Autodesk Fusion 360 part; units mm, degrees
note: some values were not read from the file. Chosen so that the rebuilt part matches the saved one: which bodies a step acts on; which face or edge a step refers to. Set by a fixed rule: which sketch regions a step uses.
(part 2 of 2)
  dimension "d542" = 3
  dimension "d543" = 3
  dimension "d544" = 3
  dimension "d545" = 3
  dimension "d571" = 15
  dimension "d572" = 30
  dimension "d573" = 15
  dimension "d574" = 30
  dimension "d575" = 30
  dimension "d576" = 5.5
  dimension "d578" = 30
  dimension "d579" = 5
  dimension "d580" = 5
  dimension "d581" = 5
  dimension "d582" = 5
  dimension "d583" = 15
  dimension "d584" = 30
  dimension "d585" = 30
  dimension "d586" = 15
  dimension "d587" = 30
  dimension "d588" = 5.5
  dimension "d591" = 30
  dimension "d592" = 5
  dimension "d593" = 5
  dimension "d594" = 5
  dimension "d595" = 5
  constraint perpendicular L3 L20
  constraint tangent A0 L2
  constraint tangent A0 L21
  constraint tangent L1 A13
  constraint tangent L21 A13
  constraint tangent A3 L3
  constraint tangent A3 L20
  constraint tangent L8 A8
  constraint tangent A8 L20
  constraint tangent L16 A782
  constraint tangent L9 A782
  constraint tangent L6 A783
  constraint tangent L9 A783
  constraint tangent L12 A784
  constraint tangent L13 A784
  constraint tangent L10 A785
  constraint tangent L13 A785
  constraint tangent L0 A786
  constraint tangent L18 A786
  constraint tangent L18 A787
  constraint tangent L19 A787
  constraint tangent L4 A788
  constraint tangent L15 A788
  constraint tangent L5 A789
  constraint tangent L4 A789
  constraint parallel L7 L23
  constraint perpendicular L6 L24
  constraint perpendicular L10 L25
  constraint tangent L25 A791
  constraint coincident L10.start A791.start
  constraint tangent L24 A792
  constraint coincident L12.end A792.end
  constraint tangent L24 A793
  constraint coincident L6.start A793.start
  constraint tangent L23 A794
  constraint coincident L16.end A794.end
  constraint parallel L3 L26
  constraint perpendicular L0 L28
  constraint tangent L28 A796
  constraint coincident L0.end A796.start
  constraint tangent L27 A797
  constraint coincident L19.start A797.end
  constraint tangent L27 A798
  constraint coincident L15.end A798.start
  constraint tangent L26 A799
  constraint coincident L5.start A799.end
  measures "d1" diameter of A12
  measures "d4" radius of A0
  measures "d5" radius of A13
  measures "d6" radius of A3
  measures "d7" radius of A8
  measures "d116" distance of A17.centre A14.centre
  measures "d152" distance of A14.centre A17.centre
  measures "d227" distance of A14.centre A17.centre
  measures "d230" distance of A14.centre A17.centre
  measures "d232" distance of L20 L21
  measures "d303" distance of A14.centre A17.centre
  measures "d305" distance of A16.centre A15.centre
  measures "d306" distance of A14.centre A17.centre
  measures "d310" distance of A14.centre A17.centre
  measures "d313" distance of A14.centre A17.centre
  measures "d319" vertical distance of A14.centre A15.centre
  measures "d448" distance of A494.centre A430.centre
  measures "d449" distance of A494.centre A430.centre
  measures "d450" distance of A494.centre A430.centre
  measures "d451" distance of A494.centre A430.centre
  measures "d452" distance of A494.centre A430.centre
  measures "d453" distance of A432.centre A473.centre
  measures "d454" distance of A430.centre A494.centre
  measures "d455" distance of A430.centre A494.centre
  measures "d456" distance of A494.centre A430.centre
  measures "d457" vertical distance of A494.centre A432.centre
  measures "d459" distance of L20 A56.centre
  measures "d460" distance of L21 A428.centre
  measures "d461" vertical distance of A53.centre A427.centre
  measures "d538" radius of A782
  measures "d539" radius of A783
  measures "d540" radius of A784
  measures "d541" radius of A785
  measures "d542" radius of A786
  measures "d543" radius of A787
  measures "d544" radius of A788
  measures "d545" radius of A789
  measures "d571" distance of A10.centre L21
  measures "d572" distance of A9.centre A10.centre
  measures "d573" distance of A6.centre L20
  measures "d574" distance of A11.centre A6.centre A430.centre
  measures "d575" distance of A9.centre A1.centre A430.centre
  measures "d576" diameter of A790
  measures "d578" distance of A11.centre A790.centre
  measures "d579" radius of A791
  measures "d580" radius of A792
  measures "d581" radius of A793
  measures "d582" radius of A794
  measures "d583" distance of A2.centre L21
  measures "d584" distance of A2.centre A4.centre
  measures "d585" distance of A5.centre A4.centre
  measures "d586" distance of A12.centre L22
  measures "d587" distance of A12.centre A7.centre
  measures "d588" diameter of A795
  measures "d591" distance of A5.centre A795.centre
  measures "d592" radius of A796
  measures "d593" radius of A797
  measures "d594" radius of A798
  measures "d595" radius of A799
extrude "Extrude1" add sketch "Sketch1" along normal blind 3 contours A0 L0 L1 A3 L2 L3 L4 L5 L6 L7 L8 A8 L9 L10 L11 L12 L13 L15 L16 L18 L19 L20 L21 A13 L22 A782 A783 A784 A785 A786 A787 A788 A789 L23 L24 L25 A791 A792 A793 A794 L26 L27 L28 A796 A797 A798 A799 | A14 A18 A26 A29 A66 A73 A87 A88 A115 A123 A124 A130 A134 A154 A174 A191 A250 A254 A306 A313 A323 A326 A328 A337 A338 A339 A340 A345 A347 A348 A364 A380 | A15 A20 A22 A27 A64 A65 A77 A83 A129 A131 A138 A159 A171 A176 A193 A200 A222 A226 A232 A234 A235 A245 A261 A277 A285 A289 A295 A310 A357 A376 A381 A385 | A16 A19 A24 A28 A68 A72 A105 A109 A121 A127 A136 A156 A158 A166 A184 A190 A247 A251 A255 A256 A263 A264 A276 A283 A293 A307 A314 A319 A320 A336 A359 A383 | A17 A21 A23 A25 A69 A86 A92 A102 A128 A133 A155 A167 A180 A182 A197 A202 A219 A220 A221 A227 A230 A241 A257 A260 A270 A279 A291 A369 A371 A386 A387 A394 | A30 A93 A126 A169 A267 A312 A316 A389 | A31 A84 A151 A163 A215 A290 A362 A395 | A32 A104 A157 A195 A233 A294 A365 A374 | A33 A82 A116 A147 A262 A288 A324 A325 | A34 A71 A120 A185 A259 A265 A309 A317 | A35 A90 A140 A173 A206 A210 A212 A213 | A36 A67 A118 A139 A207 A208 A297 A299 | A37 A108 A114 A122 A209 A211 A296 A300 | A38 A96 A150 A204 A266 A382 A384 A390 | A39 A97 A144 A179 A268 A287 A366 A373 | A40 A91 A145 A177 A282 A358 A372 A379 | A41 A70 A132 A188 A253 A305 A311 A333 | A42 A89 A189 A196 A273 A274 A286 A363 | A43 A79 A153 A199 A301 A302 A341 A342 | A44 A95 A152 A201 A303 A304 A331 A349 | A45 A80 A141 A175 A284 A308 A315 A344 | A46 A103 A119 A178 A223 A321 A329 A355 | A47 A106 A165 A203 A249 A281 A334 A346 | A48 A107 A162 A192 A236 A278 A327 A354 | A49 A78 A187 A198 A280 A332 A335 A367 | A50 A63 A117 A142 A318 A322 A330 A343 | A51 A81 A183 A186 A214 A217 A298 A353 | A52 A75 A135 A143 A224 A225 A231 A350 | A53 A76 A137 A146 A216 A239 A351 A352 | A54 A99 A110 A112 A246 A361 A377 A396 | A55 A101 A113 A168 A218 A237 A240 A388 | A56 A98 A111 A164 A229 A370 A392 A397 | A57 A94 A125 A205 A228 A244 A356 A391 | A58 A74 A148 A170 A242 A243 A252 A275 | A59 A85 A149 A161 A258 A269 A360 A375 | A60 A100 A181 A194 A272 A292 A368 A378 | A61 A62 A160 A172 A238 A248 A271 A393 | A398 A416 A419 A421 A569 A574 A645 A747 | A399 A409 A575 A644 A658 A661 A671 A775 | A400 A402 A404 A406 A418 A420 A426 A572 | A401 A403 A405 A411 A412 A423 A571 A776 | A407 A408 A422 A570 A573 A641 A646 A748 | A410 A414 A417 A750 A774 A777 A779 A781 | A413 A424 A567 A576 A640 A751 A752 A780 | A415 A425 A568 A649 A653 A749 A753 A778 | A427 A435 A437 A438 A551 A694 A721 A728 | A428 A431 A517 A519 A690 A692 A706 A731 | A429 A443 A445 A452 A542 A561 A718 A744 | A430 A434 A442 A447 A449 A451 A472 A508 A521 A525 A531 A540 A541 A545 A548 A550 A563 A566 A678 A681 A691 A696 A701 A703 A708 A712 A715 A720 A723 A724 A735 A743 | A432 A444 A446 A471 A480 A484 A489 A490 A493 A495 A511 A512 A515 A520 A530 A533 A579 A597 A598 A682 A683 A685 A693 A697 A707 A711 A716 A719 A729 A732 A733 A737 | A433 A440 A448 A677 A722 A734 A742 A746 | A436 A513 A534 A535 A537 A679 A686 A738 | A439 A441 A547 A553 A554 A555 A556 A560 | A450 A475 A498 A522 A689 A698 A709 A726 | A453 A454 A462 A465 A651 A659 A664 A673 | A455 A458 A464 A467 A470 A543 A549 A565 | A456 A457 A469 A656 A657 A663 A668 A669 | A459 A463 A466 A559 A643 A648 A660 A670 | A460 A544 A546 A552 A557 A558 A562 A564 | A461 A468 A652 A662 A666 A672 A674 A675 | A473 A476 A477 A485 A496 A497 A501 A503 A504 A518 A523 A527 A529 A532 A538 A582 A586 A588 A594 A599 A684 A688 A699 A700 A704 A705 A710 A713 A714 A727 A730 A745 | A474 A487 A502 A578 A589 A619 A631 A639 | A478 A486 A506 A516 A536 A581 A587 A601 | A479 A481 A483 A505 A577 A580 A627 A635 | A482 A491 A500 A526 A528 A583 A592 A600 | A488 A499 A584 A585 A590 A591 A595 A596 | A492 A507 A509 A510 A514 A524 A539 A687 | A494 A602 A603 A604 A605 A606 A607 A609 A610 A612 A613 A617 A618 A621 A622 A623 A624 A626 A629 A630 A633 A634 A636 A637 A638 A702 A758 A759 A761 A767 A769 A771 | A593 A608 A611 A616 A620 A628 A757 A772 | A614 A615 A632 A755 A756 A762 A763 A766 | A625 A754 A760 A764 A765 A768 A770 A773 | A642 A647 A650 A654 A655 A665 A667 A676 | A680 A695 A717 A725 A736 A739 A740 A741 | A790 | A795 makes body 1
sketch "Sketch2" plane through (0, 3, 0) normal (0, 1, 0) x (-1, 0, 0)
  circle A0 centre (-15, -105) radius 2.75
  circle A1 centre (-184, -165) radius 2.75
  circle A2 centre (-184, -135) radius 2.75
  circle A3 centre (-184, -105) radius 2.75
  circle A4 centre (-15, -15) radius 2.75
  circle A5 centre (-184, -45) radius 2.75
  circle A6 centre (-15, -135) radius 2.75
  circle A7 centre (-15, -165) radius 2.75
  circle A8 centre (-15, -45) radius 2.75
  circle A9 centre (-184, -15) radius 2.75
  line L0 (-28, -115) -> (-5, -115)
  line L1 (0, -110) -> (0, -70)
  line L2 (-5, -65) -> (-28, -65)
  line L3 (-31, -62) -> (-31, -58)
  line L4 (-28, -55) -> (-5, -55)
  line L5 (0, -50) -> (0, -10)
  arc A10 (0, -10) -> (-10, 0) centre (-10, -10) ccw
  line L6 (-10, 0) -> (-189, 0)
  arc A11 (-189, 0) -> (-199, -10) centre (-189, -10) ccw
  line L7 (-199, -10) -> (-199, -50)
  line L8 (-194, -55) -> (-171, -55)
  line L9 (-168, -58) -> (-168, -62)
  line L10 (-171, -65) -> (-194, -65)
  line L11 (-194, -115) -> (-171, -115)
  line L12 (-168, -118) -> (-168, -122)
  line L13 (-171, -125) -> (-194, -125)
  line L14 (-199, -130) -> (-199, -170)
  arc A12 (-199, -170) -> (-189, -180) centre (-189, -170) ccw
  line L15 (-189, -180) -> (-10, -180)
  arc A13 (-10, -180) -> (0, -170) centre (-10, -170) ccw
  line L16 (0, -170) -> (0, -130)
  line L17 (-5, -125) -> (-28, -125)
  line L18 (-31, -122) -> (-31, -118)
  circle A14 centre (-50, -40) radius 10
  circle A15 centre (-50, -140) radius 10
  circle A16 centre (-110, -140) radius 10
  circle A17 centre (-110, -90) radius 12.5
  circle A18 centre (-110, -40) radius 10
  circle A19 centre (-160, -90) radius 1.75
  circle A20 centre (-150, -90) radius 1.75
  circle A21 centre (-140, -90) radius 1.75
  circle A22 centre (-130, -90) radius 1.75
  circle A23 centre (-90, -90) radius 1.75
  circle A24 centre (-80, -90) radius 1.75
  circle A25 centre (-70, -90) radius 1.75
  circle A26 centre (-60, -90) radius 1.75
  circle A27 centre (-50, -90) radius 1.75
  line L19 (-10, 0) -> (-189, 0)
  line L20 (0, -60) -> (0, -30)
  line L21 (0, -142) -> (0, -128.1084)
  line L22 (-10, -180) -> (-189, -180)
  circle A28 centre (-99.8, -157.5) radius 1.75
  circle A29 centre (-122.8, -157.5) radius 1.75
  circle A30 centre (-121.5, -122.5) radius 1.75
  circle A31 centre (-98.5, -122.5) radius 1.75
  arc A32 (-168, -58) -> (-171, -55) centre (-171, -58) ccw
  arc A33 (-171, -65) -> (-168, -62) centre (-171, -62) ccw
  arc A34 (-168, -118) -> (-171, -115) centre (-171, -118) ccw
  arc A35 (-171, -125) -> (-168, -122) centre (-171, -122) ccw
  arc A36 (-31, -122) -> (-28, -125) centre (-28, -122) ccw
  arc A37 (-28, -115) -> (-31, -118) centre (-28, -118) ccw
  arc A38 (-31, -62) -> (-28, -65) centre (-28, -62) ccw
  arc A39 (-28, -55) -> (-31, -58) centre (-28, -58) ccw
  circle A40 centre (-98.5, -57.5) radius 1.75
  circle A41 centre (-120.2, -22.5) radius 1.75
  circle A42 centre (-97.2, -22.5) radius 1.75
  circle A43 centre (-121.5, -57.5) radius 1.75
  arc A44 (-199, -50) -> (-194, -55) centre (-194, -50) ccw
  arc A45 (-194, -65) -> (-199, -70) centre (-194, -70) ccw
  line L23 (-199, -70) -> (-199, -110)
  arc A46 (-199, -110) -> (-194, -115) centre (-194, -110) ccw
  arc A47 (-194, -125) -> (-199, -130) centre (-194, -130) ccw
  arc A48 (0, -130) -> (-5, -125) centre (-5, -130) ccw
  arc A49 (-5, -115) -> (0, -110) centre (-5, -110) ccw
  arc A50 (0, -70) -> (-5, -65) centre (-5, -70) ccw
  arc A51 (-5, -55) -> (0, -50) centre (-5, -50) ccw
  point P0 (-63, -24)
  point P1 (-63, -24)
  point P2 (-64.3, -156)
  point P3 (-63, -121.74)
  dimension "d468" = 20
  dimension "d472" = 20
  dimension "d477" = 20
  dimension "d478" = 25
  dimension "d479" = 20
  dimension "d480" = 50
  dimension "d483" = 3.5
  dimension "d486" = 30
  dimension "d487" = 0
  dimension "d488" = 3.5
  dimension "d491" = 40
  dimension "d492" = 0
  dimension "d508" = 50
  dimension "d509" = 50
  dimension "d513" = 40
  dimension "d514" = 40
  dimension "d515" = 3.5
  dimension "d516" = 3.5
  dimension "d517" = 3.5
  dimension "d518" = 3.5
  dimension "d519" = 23
  dimension "d520" = 23
  dimension "d521" = 35
  dimension "d522" = 35
  dimension "d556" = 3.5
  dimension "d557" = 3.5
  dimension "d558" = 3.5
  dimension "d559" = 3.5
  dimension "d560" = 23
  dimension "d561" = 23
  dimension "d562" = 35
  dimension "d563" = 35
  dimension "d564" = 11.5
  dimension "d565" = 17.5
  dimension "d567" = 11.5
  dimension "d568" = 17.5
  measures "d468" diameter of A14
  measures "d472" diameter of A15
  measures "d477" diameter of A16
  measures "d478" diameter of A17
  measures "d479" diameter of A18
  measures "d480" distance of A17.centre A18.centre
  measures "d483" diameter of A19
  measures "d488" diameter of A23
  measures "d508" distance of A14.centre L20
  measures "d509" distance of A15.centre L21
  measures "d513" distance of A14.centre L19
  measures "d514" distance of A15.centre L22
  measures "d515" diameter of A28
  measures "d516" diameter of A29
  measures "d517" diameter of A31
  measures "d518" diameter of A30
  measures "d519" distance of A28.centre A29.centre
  measures "d520" horizontal distance of A30.centre A31.centre
  measures "d521" vertical distance of A29.centre A30.centre
  measures "d522" vertical distance of A28.centre A31.centre
  measures "d556" diameter of A40
  measures "d557" diameter of A43
  measures "d558" diameter of A42
  measures "d559" diameter of A41
  measures "d560" distance of A40.centre A43.centre
  measures "d561" horizontal distance of A42.centre A41.centre
  measures "d562" vertical distance of A43.centre A41.centre
  measures "d563" vertical distance of A40.centre A42.centre
  measures "d564" horizontal distance of A16.centre A30.centre
  measures "d565" vertical distance of A16.centre A28.centre
  measures "d567" horizontal distance of A18.centre A43.centre
  measures "d568" vertical distance of A18.centre A43.centre
extrude "Extrude2" cut sketch "Sketch2" against normal blind 3 contours A14 bodies 1
extrude "Extrude4" cut sketch "Sketch2" against normal blind 3 contours A15 bodies 1
extrude "Extrude5" cut sketch "Sketch2" against normal blind 3 contours A16 | A17 | A18 bodies 1
extrude "Extrude6" cut sketch "Sketch2" against normal blind 3 contours A19 | A20 | A21 | A22 | A23 | A24 | A25 | A26 | A27 bodies 1
extrude "Extrude7" add sketch "Sketch2" against normal blind 3 contours A14 bodies 1
extrude "Extrude8" add sketch "Sketch2" against normal blind 3 contours A15 bodies 1
extrude "Extrude9" cut sketch "Sketch2" against normal blind 3 contours A14 | A15 | A28 | A29 | A30 | A31 bodies 1
extrude "Extrude10" cut sketch "Sketch1" along normal blind 3 contours A14 A18 A26 A29 A66 A73 A87 A88 A115 A123 A124 A130 A134 A154 A174 A191 A250 A254 A306 A313 A323 A326 A328 A337 A338 A339 A340 A345 A347 A348 A364 A380 | A15 A20 A22 A27 A64 A65 A77 A83 A129 A131 A138 A159 A171 A176 A193 A200 A222 A226 A232 A234 A235 A245 A261 A277 A285 A289 A295 A310 A357 A376 A381 A385 | A16 A19 A24 A28 A68 A72 A105 A109 A121 A127 A136 A156 A158 A166 A184 A190 A247 A251 A255 A256 A263 A264 A276 A283 A293 A307 A314 A319 A320 A336 A359 A383 | A17 A21 A23 A25 A69 A86 A92 A102 A128 A133 A155 A167 A180 A182 A197 A202 A219 A220 A221 A227 A230 A241 A257 A260 A270 A279 A291 A369 A371 A386 A387 A394 | A30 A93 A126 A169 A267 A312 A316 A389 | A31 A84 A151 A163 A215 A290 A362 A395 | A32 A104 A157 A195 A233 A294 A365 A374 | A33 A82 A116 A147 A262 A288 A324 A325 | A34 A71 A120 A185 A259 A265 A309 A317 | A35 A90 A140 A173 A206 A210 A212 A213 | A36 A67 A118 A139 A207 A208 A297 A299 | A37 A108 A114 A122 A209 A211 A296 A300 | A38 A96 A150 A204 A266 A382 A384 A390 | A39 A97 A144 A179 A268 A287 A366 A373 | A40 A91 A145 A177 A282 A358 A372 A379 | A41 A70 A132 A188 A253 A305 A311 A333 | A42 A89 A189 A196 A273 A274 A286 A363 | A43 A79 A153 A199 A301 A302 A341 A342 | A44 A95 A152 A201 A303 A304 A331 A349 | A45 A80 A141 A175 A284 A308 A315 A344 | A46 A103 A119 A178 A223 A321 A329 A355 | A47 A106 A165 A203 A249 A281 A334 A346 | A48 A107 A162 A192 A236 A278 A327 A354 | A49 A78 A187 A198 A280 A332 A335 A367 | A50 A63 A117 A142 A318 A322 A330 A343 | A51 A81 A183 A186 A214 A217 A298 A353 | A52 A75 A135 A143 A224 A225 A231 A350 | A53 A76 A137 A146 A216 A239 A351 A352 | A54 A99 A110 A112 A246 A361 A377 A396 | A55 A101 A113 A168 A218 A237 A240 A388 | A56 A98 A111 A164 A229 A370 A392 A397 | A57 A94 A125 A205 A228 A244 A356 A391 | A58 A74 A148 A170 A242 A243 A252 A275 | A59 A85 A149 A161 A258 A269 A360 A375 | A60 A100 A181 A194 A272 A292 A368 A378 | A61 A62 A160 A172 A238 A248 A271 A393 | A398 A416 A419 A421 A569 A574 A645 A747 | A399 A409 A575 A644 A658 A661 A671 A775 | A400 A402 A404 A406 A418 A420 A426 A572 | A401 A403 A405 A411 A412 A423 A571 A776 | A407 A408 A422 A570 A573 A641 A646 A748 | A410 A414 A417 A750 A774 A777 A779 A781 | A413 A424 A567 A576 A640 A751 A752 A780 | A415 A425 A568 A649 A653 A749 A753 A778 | A427 A435 A437 A438 A551 A694 A721 A728 | A428 A431 A517 A519 A690 A692 A706 A731 | A429 A443 A445 A452 A542 A561 A718 A744 | A430 A434 A442 A447 A449 A451 A472 A508 A521 A525 A531 A540 A541 A545 A548 A550 A563 A566 A678 A681 A691 A696 A701 A703 A708 A712 A715 A720 A723 A724 A735 A743 | A432 A444 A446 A471 A480 A484 A489 A490 A493 A495 A511 A512 A515 A520 A530 A533 A579 A597 A598 A682 A683 A685 A693 A697 A707 A711 A716 A719 A729 A732 A733 A737 | A433 A440 A448 A677 A722 A734 A742 A746 | A436 A513 A534 A535 A537 A679 A686 A738 | A439 A441 A547 A553 A554 A555 A556 A560 | A450 A475 A498 A522 A689 A698 A709 A726 | A453 A454 A462 A465 A651 A659 A664 A673 | A455 A458 A464 A467 A470 A543 A549 A565 | A456 A457 A469 A656 A657 A663 A668 A669 | A459 A463 A466 A559 A643 A648 A660 A670 | A460 A544 A546 A552 A557 A558 A562 A564 | A461 A468 A652 A662 A666 A672 A674 A675 | A473 A476 A477 A485 A496 A497 A501 A503 A504 A518 A523 A527 A529 A532 A538 A582 A586 A588 A594 A599 A684 A688 A699 A700 A704 A705 A710 A713 A714 A727 A730 A745 | A474 A487 A502 A578 A589 A619 A631 A639 | A478 A486 A506 A516 A536 A581 A587 A601 | A479 A481 A483 A505 A577 A580 A627 A635 | A482 A491 A500 A526 A528 A583 A592 A600 | A488 A499 A584 A585 A590 A591 A595 A596 | A492 A507 A509 A510 A514 A524 A539 A687 | A494 A602 A603 A604 A605 A606 A607 A609 A610 A612 A613 A617 A618 A621 A622 A623 A624 A626 A629 A630 A633 A634 A636 A637 A638 A702 A758 A759 A761 A767 A769 A771 | A593 A608 A611 A616 A620 A628 A757 A772 | A614 A615 A632 A755 A756 A762 A763 A766 | A625 A754 A760 A764 A765 A768 A770 A773 | A642 A647 A650 A654 A655 A665 A667 A676 | A680 A695 A717 A725 A736 A739 A740 A741 bodies 1
sketch "Sketch3" plane through (99.5, 0, -90) normal (0, 1, 0) x (1, 0, 0)
  line L0 (68.5, 90) -> (73.5, 90)
  line L1 (73.5, 90) -> (73.5, -90)
  line L2 (73.5, -90) -> (68.5, -90)
  line L3 (68.5, -90) -> (68.5, 90)
  line L4 (99.5, 60) -> (99.5, 25)
  line L5 (-68.5, 90) -> (-73.5, 90)
  line L6 (-73.5, 90) -> (-73.5, -90)
  line L7 (-73.5, -90) -> (-68.5, -90)
  line L8 (-68.5, -90) -> (-68.5, 90)
  line L9 (-99.5, 60) -> (-99.5, 22)
  dimension "d531" = 5
  dimension "d532" = 31
  dimension "d533" = 5
  dimension "d534" = 31
  constraint horizontal L0
  constraint vertical L1
  constraint horizontal L2
  constraint vertical L3
  constraint horizontal L5
  constraint vertical L6
  constraint horizontal L7
  constraint vertical L8
  measures "d531" distance of L1 L3
  measures "d532" distance of L3 L4
  measures "d533" distance of L6 L8
  measures "d534" distance of L8 L9
extrude "Extrude11" cut sketch "Sketch3" along normal blind 2 bodies 1
extrude "Extrude12" cut sketch "Sketch2" against normal blind 3 contours A28 | A29 | A30 | A31 | A40 | A41 | A42 | A43 bodies 1
extrude "Extrude13" cut sketch "Sketch1" along normal blind 3 contours A790 | A795 bodies 1
split "Split1" by plane through (168, 0, -118) normal (1, 0, 0) bodies 1 makes body 2 at (172.9668, 3, -23.8898) makes body 3 at (194.672, 3, -85.6235) makes body 4 at (172.9668, 3, -156.1102)
split "Split2" by plane through (31, 0, -118) normal (-1, 0, 0) bodies 1 makes body 5 at (4.328, 3, -85.6235) makes body 6 at (26.0332, 3, -156.1102) makes body 7 at (26.0332, 3, -23.8898)
move_body "Move1" bodies 2 3 4 to x (0, 1, 0) y (-1, 0, 0) z (0, 0, 1) at (171, -168, 0)
move_body "Move2" bodies 7 5 6 to x (0, -1, 0) y (1, 0, 0) z (0, 0, 1) at (28, 31, 0)
extrude "Extrude3" [suppressed]

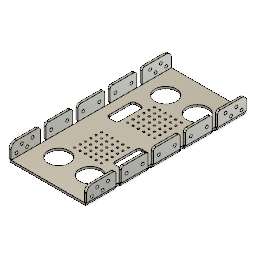
design "Trunk Bottom 4mm"
Autodesk Fusion 360 part; units mm, degrees
sketch "Sketch1" plane through (0, 0, 0) normal (0, 1, 0) x (1, 0, 0)
  line L0 (10, 0) -> (189, 0)
  line L1 (189, 300) -> (10, 300)
  circle A0 centre (184, 165) radius 2.75
  circle A1 centre (184, 135) radius 2.75
  circle A2 centre (184, 195) radius 2.75
  circle A3 centre (184, 105) radius 2.75
  arc A4 (10, 300) -> (0, 290) centre (10, 290) ccw
  arc A5 (199, 290) -> (189, 300) centre (189, 290) ccw
  arc A6 (0, 10) -> (10, 0) centre (10, 10) ccw
  arc A7 (189, 0) -> (199, 10) centre (189, 10) ccw
  circle A8 centre (184, 225) radius 2.75
  line L2 (199, 232.541) -> (199, 232)
  line L3 (199, 202) -> (199, 215)
  line L4 (199, 282) -> (199, 290)
  line L5 (194, 175) -> (171, 175)
  line L6 (171, 185) -> (194, 185)
  line L7 (168, 178) -> (168, 182)
  line L8 (194, 115) -> (171, 115)
  line L9 (171, 125) -> (194, 125)
  line L10 (168, 118) -> (168, 122)
  line L11 (0, 290) -> (0, 270)
  line L12 (0, 68.1084) -> (0, 68)
  line L13 (0, 30) -> (0, 10)
  line L14 (199, 10) -> (199, 30)
  line L15 (199, 85) -> (199, 98)
  line L16 (0, 52) -> (0, 52.1084)
  line L17 (0, 112) -> (0, 112.1084)
  line L18 (0, 142) -> (0, 142.1084)
  line L19 (0, 172) -> (0, 172.1084)
  line L20 (0, 202) -> (0, 202.1084)
  line L21 (0, 232) -> (0, 232.1084)
  line L22 (0, 262) -> (0, 262.1084)
  circle A9 centre (15, 105) radius 2.75
  circle A10 centre (15, 135) radius 2.75
  circle A11 centre (15, 165) radius 2.75
  circle A12 centre (15, 195) radius 2.75
  circle A13 centre (15, 225) radius 2.75
  line L23 (5, 115) -> (28, 115)
  line L24 (28, 125) -> (5, 125)
  line L25 (31, 118) -> (31, 122)
  line L26 (28, 185) -> (5, 185)
  line L27 (5, 175) -> (28, 175)
  line L28 (31, 178) -> (31, 182)
  circle A14 centre (10, 280) radius 2.75
  circle A15 centre (20, 270) radius 2.75
  circle A16 centre (20, 290) radius 2.75
  circle A17 centre (20, 30) radius 2.75
  circle A18 centre (10, 20) radius 2.75
  circle A19 centre (20, 10) radius 2.75
  circle A20 centre (179, 10) radius 2.75
  circle A21 centre (189, 20) radius 2.75
  circle A22 centre (179, 30) radius 2.75
  circle A23 centre (179, 270) radius 2.75
  circle A24 centre (189, 280) radius 2.75
  circle A25 centre (179, 290) radius 2.75
  circle A26 centre (70, 90) radius 1.75
  circle A27 centre (129, 210) radius 1.75
  line L29 (199, 270) -> (199, 282)
  line L30 (199, 202) -> (199, 188)
  line L31 (135, 140) -> (145, 140)
  line L32 (150, 135) -> (150, 95)
  line L33 (145, 90) -> (135, 90)
  line L34 (130, 95) -> (130, 135)
  arc A28 (135, 140) -> (130, 135) centre (135, 135) ccw
  arc A29 (150, 135) -> (145, 140) centre (145, 135) ccw
  arc A30 (145, 90) -> (150, 95) centre (145, 95) ccw
  arc A31 (130, 95) -> (135, 90) centre (135, 95) ccw
  line L35 (64, 160) -> (54, 160)
  line L36 (49, 165) -> (49, 205)
  line L37 (54, 210) -> (64, 210)
  line L38 (69, 205) -> (69, 165)
  arc A32 (54, 210) -> (49, 205) centre (54, 205) ccw
  arc A33 (49, 165) -> (54, 160) centre (54, 165) ccw
  arc A34 (64, 160) -> (69, 165) centre (64, 165) ccw
  arc A35 (69, 205) -> (64, 210) centre (64, 205) ccw
  circle A36 centre (70, 50) radius 20
  circle A37 centre (129, 50) radius 20
  circle A38 centre (70, 250) radius 20
  circle A39 centre (129, 250) radius 20
  arc A40 (31, 182) -> (28, 185) centre (28, 182) ccw
  arc A41 (28, 175) -> (31, 178) centre (28, 178) ccw
  arc A42 (31, 122) -> (28, 125) centre (28, 122) ccw
  arc A43 (28, 115) -> (31, 118) centre (28, 118) ccw
  line L39 (0, 112) -> (0, 85)
  arc A44 (171, 125) -> (168, 122) centre (171, 122) ccw
  arc A45 (168, 118) -> (171, 115) centre (171, 118) ccw
  arc A46 (171, 185) -> (168, 182) centre (171, 182) ccw
  arc A47 (168, 178) -> (171, 175) centre (171, 178) ccw
  circle A48 centre (15, 75) radius 2.75
  line L40 (28, 245) -> (5, 245)
  line L41 (5, 235) -> (28, 235)
  arc A49 (28, 235) -> (31, 238) centre (28, 238) ccw
  line L42 (31, 238) -> (31, 242)
  arc A50 (31, 242) -> (28, 245) centre (28, 242) ccw
  line L43 (28, 65) -> (5, 65)
  line L44 (5, 55) -> (28, 55)
  arc A51 (28, 55) -> (31, 58) centre (28, 58) ccw
  line L45 (31, 58) -> (31, 62)
  arc A52 (31, 62) -> (28, 65) centre (28, 62) ccw
  line L46 (0, 30) -> (0, 54.7325)
  line L47 (0, 54.7325) -> (0, 50)
  line L48 (0, 70) -> (0, 85)
  line L49 (0, 112) -> (0, 110)
  line L50 (0, 130) -> (0, 145)
  line L51 (0, 145) -> (0, 170)
  line L52 (0, 190) -> (0, 230)
  line L53 (0, 250) -> (0, 270)
  circle A53 centre (184, 75) radius 2.75
  arc A54 (5, 55) -> (0, 50) centre (5, 50) ccw
  arc A55 (0, 70) -> (5, 65) centre (5, 70) ccw
  arc A56 (5, 115) -> (0, 110) centre (5, 110) ccw
  arc A57 (0, 130) -> (5, 125) centre (5, 130) ccw
  arc A58 (5, 175) -> (0, 170) centre (5, 170) ccw
  arc A59 (0, 190) -> (5, 185) centre (5, 190) ccw
  arc A60 (5, 235) -> (0, 230) centre (5, 230) ccw
  arc A61 (0, 250) -> (5, 245) centre (5, 250) ccw
  line L54 (194, 55) -> (171, 55)
  line L55 (171, 65) -> (194, 65)
  arc A62 (171, 65) -> (168, 62) centre (171, 62) ccw
  arc A63 (168, 58) -> (171, 55) centre (171, 58) ccw
  line L56 (168, 58) -> (168, 62)
  line L57 (171, 245) -> (194, 245)
  line L58 (194, 235) -> (171, 235)
  arc A64 (168, 238) -> (171, 235) centre (171, 238) ccw
  line L59 (168, 238) -> (168, 242)
  arc A65 (171, 245) -> (168, 242) centre (171, 242) ccw
  line L60 (199, 270) -> (199, 250)
  line L61 (199, 230) -> (199, 215)
  line L62 (199, 215) -> (199, 190)
  line L63 (199, 170) -> (199, 130)
  line L64 (199, 110) -> (199, 98)
  line L65 (199, 85) -> (199, 70)
  line L66 (199, 50) -> (199, 30)
  arc A66 (199, 50) -> (194, 55) centre (194, 50) ccw
  arc A67 (194, 65) -> (199, 70) centre (194, 70) ccw
  arc A68 (199, 110) -> (194, 115) centre (194, 110) ccw
  arc A69 (194, 125) -> (199, 130) centre (194, 130) ccw
  arc A70 (199, 170) -> (194, 175) centre (194, 170) ccw
  arc A71 (194, 185) -> (199, 190) centre (194, 190) ccw
  arc A72 (199, 230) -> (194, 235) centre (194, 230) ccw
  arc A73 (194, 245) -> (199, 250) centre (194, 250) ccw
  circle A74 centre (10, 260) radius 2.75
  circle A75 centre (189, 260) radius 2.75
  circle A76 centre (189, 40) radius 2.75
  circle A77 centre (10, 40) radius 2.75
  circle A78 centre (119, 210) radius 1.75
  circle A79 centre (109, 210) radius 1.75
  circle A80 centre (99, 210) radius 1.75
  circle A81 centre (129, 200) radius 1.75
  circle A82 centre (119, 200) radius 1.75
  circle A83 centre (109, 200) radius 1.75
  circle A84 centre (99, 200) radius 1.75
  circle A85 centre (129, 190) radius 1.75
  circle A86 centre (119, 190) radius 1.75
  circle A87 centre (109, 190) radius 1.75
  circle A88 centre (99, 190) radius 1.75
  circle A89 centre (129, 180) radius 1.75
  circle A90 centre (119, 180) radius 1.75
  circle A91 centre (109, 180) radius 1.75
  circle A92 centre (99, 180) radius 1.75
  circle A93 centre (129, 170) radius 1.75
  circle A94 centre (119, 170) radius 1.75
  circle A95 centre (109, 170) radius 1.75
  circle A96 centre (99, 170) radius 1.75
  circle A97 centre (119, 220) radius 1.75
  circle A98 centre (129, 220) radius 1.75
  circle A99 centre (99, 220) radius 1.75
  circle A100 centre (109, 220) radius 1.75
  circle A101 centre (89, 210) radius 1.75
  circle A102 centre (89, 220) radius 1.75
  circle A103 centre (89, 180) radius 1.75
  circle A104 centre (89, 200) radius 1.75
  circle A105 centre (89, 190) radius 1.75
  circle A106 centre (89, 170) radius 1.75
  circle A107 centre (79, 210) radius 1.75
  circle A108 centre (79, 220) radius 1.75
  circle A109 centre (79, 180) radius 1.75
  circle A110 centre (79, 200) radius 1.75
  circle A111 centre (79, 190) radius 1.75
  circle A112 centre (79, 170) radius 1.75
  circle A113 centre (80, 90) radius 1.75
  circle A114 centre (90, 90) radius 1.75
  circle A115 centre (100, 90) radius 1.75
  circle A116 centre (110, 90) radius 1.75
  circle A117 centre (120, 90) radius 1.75
  circle A118 centre (70, 100) radius 1.75
  circle A119 centre (80, 100) radius 1.75
  circle A120 centre (90, 100) radius 1.75
  circle A121 centre (100, 100) radius 1.75
  circle A122 centre (110, 100) radius 1.75
  circle A123 centre (120, 100) radius 1.75
  circle A124 centre (70, 110) radius 1.75
  circle A125 centre (80, 110) radius 1.75
  circle A126 centre (90, 110) radius 1.75
  circle A127 centre (100, 110) radius 1.75
  circle A128 centre (110, 110) radius 1.75
  circle A129 centre (120, 110) radius 1.75
  circle A130 centre (70, 120) radius 1.75
  circle A131 centre (80, 120) radius 1.75
  circle A132 centre (90, 120) radius 1.75
  circle A133 centre (100, 120) radius 1.75
  circle A134 centre (110, 120) radius 1.75
  circle A135 centre (120, 120) radius 1.75
  circle A136 centre (70, 130) radius 1.75
  circle A137 centre (80, 130) radius 1.75
  circle A138 centre (90, 130) radius 1.75
  circle A139 centre (100, 130) radius 1.75
  circle A140 centre (110, 130) radius 1.75
  circle A141 centre (120, 130) radius 1.75
  circle A142 centre (120, 80) radius 1.75
  circle A143 centre (70, 80) radius 1.75
  circle A144 centre (90, 80) radius 1.75
  circle A145 centre (80, 80) radius 1.75
  circle A146 centre (110, 80) radius 1.75
  circle A147 centre (100, 80) radius 1.75
  point P0 (199, 0)
  point P1 (0, 300)
  point P2 (169, 190)
  point P3 (0, 170.1084)
  dimension "d1" = 199
  dimension "d2" = 300
  dimension "d14" = 5.5
  dimension "d21" = 5.5
  dimension "d24" = 5.5
  dimension "d25" = 5.5
  dimension "d39" = 10
  dimension "d40" = 10
  dimension "d41" = 10
  dimension "d42" = 10
  dimension "d53" = 5.5
  dimension "d139" = 5.5
  dimension "d140" = 10
  dimension "d142" = 5.5
  dimension "d144" = 20
  dimension "d145" = 5.5
  dimension "d148" = 0
  dimension "d149" = -260
  dimension "d177" = 3.5
  dimension "d178" = 70
  dimension "d179" = 90
  dimension "d180" = 3.5
  dimension "d181" = 90
  dimension "d198" = 5
  dimension "d199" = 5
  dimension "d202" = 40
  dimension "d203" = 50
  dimension "d205" = 40
  dimension "d207" = 40
  dimension "d208" = 40
  dimension "d211" = 50
  dimension "d212" = 50
  dimension "d232" = 3
  dimension "d233" = 3
  dimension "d234" = 3
  dimension "d235" = 3
  dimension "d246" = 3
  dimension "d247" = 3
  dimension "d248" = 3
  dimension "d249" = 3
  dimension "d258" = 75
  dimension "d259" = 30
  dimension "d260" = 30
  dimension "d261" = 30
  dimension "d262" = 30
  dimension "d263" = 5.5
  dimension "d264" = 15
  dimension "d265" = 30
  dimension "d266" = 3
  dimension "d267" = 3
  dimension "d268" = 3
  dimension "d269" = 3
  dimension "d270" = 75
  dimension "d271" = 30
  dimension "d272" = 30
  dimension "d273" = 30
  dimension "d274" = 30
  dimension "d275" = 5.5
  dimension "d277" = 30
  dimension "d278" = 5
  dimension "d279" = 5
  dimension "d280" = 5
  dimension "d281" = 5
  dimension "d282" = 5
  dimension "d283" = 5
  dimension "d284" = 5
  dimension "d285" = 5
  dimension "d286" = 3
  dimension "d287" = 3
  dimension "d288" = 3
  dimension "d289" = 3
  dimension "d290" = 5
  dimension "d291" = 5
  dimension "d292" = 5
  dimension "d293" = 5
  dimension "d294" = 5
  dimension "d295" = 5
  dimension "d296" = 5
  dimension "d297" = 5
  dimension "d300" = 5.5
  dimension "d301" = 10
  dimension "d302" = 20
  dimension "d303" = 5.5
  dimension "d304" = 10
  dimension "d305" = 20
  dimension "d306" = 5.5
  dimension "d307" = 10
  dimension "d308" = 20
  dimension "d309" = 5.5
  dimension "d310" = 20
  dimension "d315" = -30
  dimension "d316" = -50
  dimension "d321" = 0
  dimension "d322" = 10
  dimension "d329" = 50
  dimension "d330" = 50
  dimension "d333" = 70
  dimension "d334" = 18
  dimension "d335" = 18
  dimension "d338" = 0
  dimension "d339" = -10
  constraint horizontal L0
  constraint vertical L14
  constraint horizontal L1
  constraint vertical L11
  constraint coincident P1 L1
  constraint coincident P1 L11
  constraint tangent L1 A4
  constraint tangent A4 L11
  constraint tangent A5 L14
  constraint tangent L1 A5
  constraint coincident origin L0
  constraint coincident origin L11
  constraint tangent L0 A6
  constraint tangent A6 L11
  constraint coincident P0 L0
  constraint coincident P0 L14
  constraint tangent L0 A7
  constraint tangent A7 L14
  constraint collinear L3 L14
  constraint vertical L2
  constraint coincident P3 L11
  constraint collinear L12 L13
  constraint parallel L11 L22
  constraint coincident L22.end L11
  constraint horizontal L31
  constraint vertical L32
  constraint horizontal L33
  constraint vertical L34
  constraint tangent L31 A28
  constraint tangent L34 A28
  constraint tangent L31 A29
  constraint tangent L32 A29
  constraint equal A28 A29
  constraint tangent L32 A30
  constraint tangent L33 A30
  constraint equal A28 A30
  constraint tangent L33 A31
  constraint tangent L34 A31
  constraint equal A28 A31
  constraint horizontal L35
  constraint vertical L36
  constraint horizontal L37
  constraint vertical L38
  constraint tangent L36 A32
  constraint tangent L37 A32
  constraint tangent L35 A33
  constraint tangent L36 A33
  constraint equal A32 A33
  constraint tangent L35 A34
  constraint tangent L38 A34
  constraint equal A32 A34
  constraint tangent L37 A35
  constraint tangent L38 A35
  constraint equal A32 A35
  constraint tangent L26 A40
  constraint tangent L28 A40
  constraint tangent L28 A41
  constraint tangent L27 A41
  constraint tangent L24 A42
  constraint tangent L25 A42
  constraint tangent L23 A43
  constraint tangent L25 A43
  constraint tangent L10 A44
  constraint tangent L9 A44
  constraint tangent L10 A45
  constraint tangent L8 A45
  constraint tangent L7 A46
  constraint tangent L6 A46
  constraint tangent L7 A47
  constraint tangent L5 A47
  constraint tangent L40 A50
  constraint tangent L42 A50
  constraint tangent A49 L42
  constraint tangent L41 A49
  constraint tangent L43 A52
  constraint tangent L45 A52
  constraint tangent L44 A51
  constraint tangent A51 L45
  constraint parallel L13 L46
  constraint perpendicular L44 L47
  constraint parallel L50 L51
  constraint perpendicular L40 L53
  constraint tangent L47 A54
  constraint coincident L44.start A54.start
  constraint tangent L48 A55
  constraint coincident L43.end A55.end
  constraint tangent L49 A56
  constraint coincident L23.start A56.start
  constraint tangent L50 A57
  constraint coincident L24.end A57.end
  constraint tangent L51 A58
  constraint coincident L27.start A58.start
  constraint tangent L52 A59
  constraint coincident L26.end A59.end
  constraint tangent L52 A60
  constraint coincident L41.start A60.start
  constraint tangent L53 A61
  constraint coincident L40.end A61.end
  constraint tangent A62 L56
  constraint tangent L55 A62
  constraint tangent A63 L56
  constraint tangent L54 A63
  constraint tangent L59 A65
  constraint tangent L57 A65
  constraint tangent A64 L59
  constraint tangent L58 A64
  constraint parallel L29 L60
  constraint parallel L15 L65
  constraint perpendicular L54 L66
  constraint tangent L66 A66
  constraint coincident L54.start A66.end
  constraint tangent L65 A67
  constraint coincident L55.end A67.start
  constraint tangent L64 A68
  constraint coincident L8.start A68.end
  constraint tangent L63 A69
  constraint coincident L9.end A69.start
  constraint tangent L63 A70
  constraint coincident L5.start A70.end
  constraint tangent L62 A71
  constraint coincident L6.end A71.start
  constraint tangent L61 A72
  constraint coincident L58.start A72.end
  constraint tangent L60 A73
  constraint coincident L57.end A73.start
  measures "d1" distance of origin P0
  measures "d2" distance of origin P1
  measures "d14" diameter of A0
  measures "d21" diameter of A1
  measures "d24" diameter of A2
  measures "d25" diameter of A3
  measures "d39" radius of A4
  measures "d40" radius of A5
  measures "d41" radius of A6
  measures "d42" radius of A7
  measures "d53" diameter of A8
  measures "d139" diameter of A14
  measures "d140" distance of L11 A14.centre
  measures "d142" diameter of A15
  measures "d144" distance of L11 A15.centre
  measures "d145" diameter of A16
  measures "d177" diameter of A27
  measures "d178" distance of L3 A27.centre
  measures "d179" distance of L1 A27.centre
  measures "d180" diameter of A26
  measures "d181" distance of L0 A26.centre
  measures "d198" radius of A28
  measures "d199" radius of A32
  measures "d202" diameter of A36
  measures "d203" distance of L0 A36.centre
  measures "d205" diameter of A37
  measures "d207" diameter of A38
  measures "d208" diameter of A39
  measures "d211" distance of L1 A39.centre
  measures "d212" distance of L1 A38.centre
  measures "d232" radius of A40
  measures "d233" radius of A41
  measures "d234" radius of A42
  measures "d235" radius of A43
  measures "d246" radius of A44
  measures "d247" radius of A45
  measures "d248" radius of A46
  measures "d249" radius of A47
  measures "d258" distance of L1 A13.centre
  measures "d259" distance of A12.centre A13.centre
  measures "d260" distance of A11.centre A12.centre
  measures "d261" distance of A10.centre A11.centre
  measures "d262" distance of A9.centre A10.centre
  measures "d263" diameter of A48
  measures "d264" distance of L39 A48.centre
  measures "d265" distance of A9.centre A48.centre
  measures "d266" radius of A50
  measures "d267" radius of A49
  measures "d268" radius of A52
  measures "d269" radius of A51
  measures "d270" distance of L1 A8.centre
  measures "d271" distance of A2.centre A8.centre
  measures "d272" distance of A0.centre A2.centre
  measures "d273" distance of A0.centre A1.centre
  measures "d274" distance of A1.centre A3.centre
  measures "d275" diameter of A53
  measures "d277" distance of A3.centre A53.centre
  measures "d278" radius of A54
  measures "d279" radius of A55
  measures "d280" radius of A56
  measures "d281" radius of A57
  measures "d282" radius of A58
  measures "d283" radius of A59
  measures "d284" radius of A60
  measures "d285" radius of A61
  measures "d286" radius of A62
  measures "d287" radius of A63
  measures "d288" radius of A65
  measures "d289" radius of A64
  measures "d290" radius of A66
  measures "d291" radius of A67
  measures "d292" radius of A68
  measures "d293" radius of A69
  measures "d294" radius of A70
  measures "d295" radius of A71
  measures "d296" radius of A72
  measures "d297" radius of A73
  measures "d300" diameter of A74
  measures "d301" distance of L53 A74.centre
  measures "d302" distance of A14.centre A74.centre
  measures "d303" diameter of A75
  measures "d304" distance of L60 A75.centre
  measures "d305" distance of A24.centre A75.centre
  measures "d306" diameter of A76
  measures "d307" distance of L66 A76.centre
  measures "d308" distance of A21.centre A76.centre
  measures "d309" diameter of A77
  measures "d310" distance of A18.centre A77.centre
  measures "d333" distance of A26.centre L39
  measures "d334" distance of L10 L32
  measures "d335" distance of L28 L36
sketch "Sketch3" plane through (0, 0, 0) normal (0, 1, 0) x (1, 0, 0)
  line L0 (173, 300) -> (168, 300)
  line L1 (168, 300) -> (168, 0)
  line L2 (168, 0) -> (173, 0)
  line L3 (173, 0) -> (173, 300)
  line L4 (31, 300) -> (26, 300)
  line L5 (26, 300) -> (26, 0)
  line L6 (26, 0) -> (31, 0)
  line L7 (31, 0) -> (31, 300)
  line L8 (0, 290) -> (0, 270)
  line L9 (199, 282) -> (199, 290)
  dimension "d152" = 5
  dimension "d154" = 5
  dimension "d155" = 31
  dimension "d215" = 31
  constraint horizontal L0
  constraint vertical L1
  constraint horizontal L2
  constraint vertical L3
  constraint horizontal L4
  constraint vertical L5
  constraint horizontal L6
  constraint vertical L7
  measures "d152" distance of L1 L3
  measures "d154" distance of L5 L7
  measures "d155" distance of L7 L8
  measures "d215" distance of L1 L9
extrude "Extrude15" add sketch "Sketch1" along normal blind 4 makes body 1
extrude "Extrude16" cut sketch "Sketch3" along normal blind 2 bodies 1
split "Split1" by plane through (168, 0, -300) normal (1, 0, 0) bodies 1 makes body 2 at (184.2083, 4, -50.7939) makes body 3 at (194.672, 4, -205.6235) makes body 4 at (194.672, 4, -145.6235) makes body 5 at (194.672, 4, -94.3765) makes body 6 at (184.2083, 4, -249.2061)
move_body "Move1" bodies 2 4 5 6 3 to x (0, 1, 0) y (-1, 0, 0) z (0, 0, 1) at (172, -168, 0)
split "Split2" by plane through (31, 0, 0) normal (-1, 0, 0) bodies 1 makes body 7 at (14.7917, 4, -249.2061) makes body 8 at (4.328, 4, -154.3765) makes body 9 at (4.328, 4, -205.6235) makes body 10 at (14.7917, 4, -50.7939) makes body 11 at (4.328, 4, -85.6235)
move_body "Move2" bodies 7 11 10 8 9 to x (0, -1, 0) y (1, 0, 0) z (0, 0, 1) at (27, 31, 0)
combine "Combine1" operation add target body 1 tool bodies 2 11 10 8 9 7 4 5 6 3
